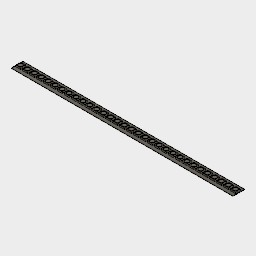
1376 NeoPixel Strip [parametric] (Autodesk Fusion 360 design; units mm, degrees)
Autodesk Fusion 360 part; units mm, degrees
sketch "pixels" plane through (0, 0, 0) normal (0, 0, 1) x (1, 0, 0)
  line L0 (0, 0) -> (224, 0)
  line L1 (224, 0) -> (224, 12)
  line L2 (224, 12) -> (0, 12)
  line L3 (0, 12) -> (0, 0)
  line L4 (0, 6) -> (224, 6) construction
  line L5 (6, 3.5) -> (1, 3.5)
  line L6 (1, 3.5) -> (1, 8.5)
  line L7 (1, 8.5) -> (6, 8.5)
  line L8 (6, 8.5) -> (6, 3.5)
  line L9 (6, 3.5) -> (1, 8.5) construction
  line L10 (1, 3.5) -> (6, 8.5) construction
  line L11 (13, 3.5) -> (8, 3.5)
  line L12 (8, 3.5) -> (8, 8.5)
  line L13 (8, 8.5) -> (13, 8.5)
  line L14 (13, 8.5) -> (13, 3.5)
  line L15 (20, 3.5) -> (15, 3.5)
  line L16 (15, 3.5) -> (15, 8.5)
  line L17 (15, 8.5) -> (20, 8.5)
  line L18 (20, 8.5) -> (20, 3.5)
  line L19 (27, 3.5) -> (22, 3.5)
  line L20 (22, 3.5) -> (22, 8.5)
  line L21 (22, 8.5) -> (27, 8.5)
  line L22 (27, 8.5) -> (27, 3.5)
  line L23 (34, 3.5) -> (29, 3.5)
  line L24 (29, 3.5) -> (29, 8.5)
  line L25 (29, 8.5) -> (34, 8.5)
  line L26 (34, 8.5) -> (34, 3.5)
  line L27 (41, 3.5) -> (36, 3.5)
  line L28 (36, 3.5) -> (36, 8.5)
  line L29 (36, 8.5) -> (41, 8.5)
  line L30 (41, 8.5) -> (41, 3.5)
  line L31 (48, 3.5) -> (43, 3.5)
  line L32 (43, 3.5) -> (43, 8.5)
  line L33 (43, 8.5) -> (48, 8.5)
  line L34 (48, 8.5) -> (48, 3.5)
  line L35 (55, 3.5) -> (50, 3.5)
  line L36 (50, 3.5) -> (50, 8.5)
  line L37 (50, 8.5) -> (55, 8.5)
  line L38 (55, 8.5) -> (55, 3.5)
  line L39 (62, 3.5) -> (57, 3.5)
  line L40 (57, 3.5) -> (57, 8.5)
  line L41 (57, 8.5) -> (62, 8.5)
  line L42 (62, 8.5) -> (62, 3.5)
  line L43 (69, 3.5) -> (64, 3.5)
  line L44 (64, 3.5) -> (64, 8.5)
  line L45 (64, 8.5) -> (69, 8.5)
  line L46 (69, 8.5) -> (69, 3.5)
  line L47 (76, 3.5) -> (71, 3.5)
  line L48 (71, 3.5) -> (71, 8.5)
  line L49 (71, 8.5) -> (76, 8.5)
  line L50 (76, 8.5) -> (76, 3.5)
  line L51 (83, 3.5) -> (78, 3.5)
  line L52 (78, 3.5) -> (78, 8.5)
  line L53 (78, 8.5) -> (83, 8.5)
  line L54 (83, 8.5) -> (83, 3.5)
  line L55 (90, 3.5) -> (85, 3.5)
  line L56 (85, 3.5) -> (85, 8.5)
  line L57 (85, 8.5) -> (90, 8.5)
  line L58 (90, 8.5) -> (90, 3.5)
  line L59 (97, 3.5) -> (92, 3.5)
  line L60 (92, 3.5) -> (92, 8.5)
  line L61 (92, 8.5) -> (97, 8.5)
  line L62 (97, 8.5) -> (97, 3.5)
  line L63 (104, 3.5) -> (99, 3.5)
  line L64 (99, 3.5) -> (99, 8.5)
  line L65 (99, 8.5) -> (104, 8.5)
  line L66 (104, 8.5) -> (104, 3.5)
  line L67 (111, 3.5) -> (106, 3.5)
  line L68 (106, 3.5) -> (106, 8.5)
  line L69 (106, 8.5) -> (111, 8.5)
  line L70 (111, 8.5) -> (111, 3.5)
  line L71 (118, 3.5) -> (113, 3.5)
  line L72 (113, 3.5) -> (113, 8.5)
  line L73 (113, 8.5) -> (118, 8.5)
  line L74 (118, 8.5) -> (118, 3.5)
  line L75 (125, 3.5) -> (120, 3.5)
  line L76 (120, 3.5) -> (120, 8.5)
  line L77 (120, 8.5) -> (125, 8.5)
  line L78 (125, 8.5) -> (125, 3.5)
  line L79 (132, 3.5) -> (127, 3.5)
  line L80 (127, 3.5) -> (127, 8.5)
  line L81 (127, 8.5) -> (132, 8.5)
  line L82 (132, 8.5) -> (132, 3.5)
  line L83 (139, 3.5) -> (134, 3.5)
  line L84 (134, 3.5) -> (134, 8.5)
  line L85 (134, 8.5) -> (139, 8.5)
  line L86 (139, 8.5) -> (139, 3.5)
  line L87 (146, 3.5) -> (141, 3.5)
  line L88 (141, 3.5) -> (141, 8.5)
  line L89 (141, 8.5) -> (146, 8.5)
  line L90 (146, 8.5) -> (146, 3.5)
  line L91 (153, 3.5) -> (148, 3.5)
  line L92 (148, 3.5) -> (148, 8.5)
  line L93 (148, 8.5) -> (153, 8.5)
  line L94 (153, 8.5) -> (153, 3.5)
  line L95 (160, 3.5) -> (155, 3.5)
  line L96 (155, 3.5) -> (155, 8.5)
  line L97 (155, 8.5) -> (160, 8.5)
  line L98 (160, 8.5) -> (160, 3.5)
  line L99 (167, 3.5) -> (162, 3.5)
  line L100 (162, 3.5) -> (162, 8.5)
  line L101 (162, 8.5) -> (167, 8.5)
  line L102 (167, 8.5) -> (167, 3.5)
  line L103 (174, 3.5) -> (169, 3.5)
  line L104 (169, 3.5) -> (169, 8.5)
  line L105 (169, 8.5) -> (174, 8.5)
  line L106 (174, 8.5) -> (174, 3.5)
  line L107 (181, 3.5) -> (176, 3.5)
  line L108 (176, 3.5) -> (176, 8.5)
  line L109 (176, 8.5) -> (181, 8.5)
  line L110 (181, 8.5) -> (181, 3.5)
  line L111 (188, 3.5) -> (183, 3.5)
  line L112 (183, 3.5) -> (183, 8.5)
  line L113 (183, 8.5) -> (188, 8.5)
  line L114 (188, 8.5) -> (188, 3.5)
  line L115 (195, 3.5) -> (190, 3.5)
  line L116 (190, 3.5) -> (190, 8.5)
  line L117 (190, 8.5) -> (195, 8.5)
  line L118 (195, 8.5) -> (195, 3.5)
  line L119 (202, 3.5) -> (197, 3.5)
  line L120 (197, 3.5) -> (197, 8.5)
  line L121 (197, 8.5) -> (202, 8.5)
  line L122 (202, 8.5) -> (202, 3.5)
  line L123 (209, 3.5) -> (204, 3.5)
  line L124 (204, 3.5) -> (204, 8.5)
  line L125 (204, 8.5) -> (209, 8.5)
  line L126 (209, 8.5) -> (209, 3.5)
  line L127 (216, 3.5) -> (211, 3.5)
  line L128 (211, 3.5) -> (211, 8.5)
  line L129 (211, 8.5) -> (216, 8.5)
  line L130 (216, 8.5) -> (216, 3.5)
  line L131 (223, 3.5) -> (218, 3.5)
  line L132 (218, 3.5) -> (218, 8.5)
  line L133 (218, 8.5) -> (223, 8.5)
  line L134 (223, 8.5) -> (223, 3.5)
  point P0 (3.5, 6)
  dimension "d4" = 224
  dimension "d5" = 12
  dimension "d6" = 5
  dimension "d7" = 5
  dimension "d8" = 3.5
  dimension "d11" = 7
  dimension "d12" = 0
  measures "d4" distance of L0.start L0.end
  measures "d5" distance of L0.start L2.end
  measures "d6" distance of L6.end L7.end
  measures "d7" distance of L5.end L6.end
  measures "d8" distance of L3 P0
extrude "Extrude1" add sketch "pixels" along normal blind 0.34 contours L0 L1 L2 L3 | L5 L6 L7 L8 | L11 L12 L13 L14 | L15 L16 L17 L18 | L19 L20 L21 L22 | L23 L24 L25 L26 | L27 L28 L29 L30 | L31 L32 L33 L34 | L35 L36 L37 L38 | L39 L40 L41 L42 | L43 L44 L45 L46 | L47 L48 L49 L50 | L51 L52 L53 L54 | L55 L56 L57 L58 | L59 L60 L61 L62 | L63 L64 L65 L66 | L67 L68 L69 L70 | L71 L72 L73 L74 | L75 L76 L77 L78 | L79 L80 L81 L82 | L83 L84 L85 L86 | L87 L88 L89 L90 | L91 L92 L93 L94 | L95 L96 L97 L98 | L99 L100 L101 L102 | L103 L104 L105 L106 | L107 L108 L109 L110 | L111 L112 L113 L114 | L115 L116 L117 L118 | L119 L120 L121 L122 | L123 L124 L125 L126 | L127 L128 L129 L130 | L131 L132 L133 L134
extrude "Extrude2" add sketch "pixels" along normal blind 1.4 from surface at 0.34 contours L5 L6 L7 L8
pattern_linear "R-Pattern2" count 32 spacing 7 along (1, 0, 0) of "Extrude2"
sketch "circles" plane through (0, 0, 1.74) normal (0, 0, 1) x (-1, 0, 0)
  line L0 (-6, -8.5) -> (-1, -8.5)
  line L1 (-1, -8.5) -> (-1, -3.5)
  line L2 (-1, -3.5) -> (-6, -3.5)
  line L3 (-6, -3.5) -> (-6, -8.5)
  line L4 (-1, -6) -> (-6, -6) construction
  line L5 (-3.5, -8.5) -> (-3.5, -3.5) construction
  circle A0 centre (-3.5, -6) radius 2
  dimension "d20" = 4
  measures "d20" diameter of A0
extrude "Extrude3" cut sketch "circles" against normal blind 0.2 contours A0
pattern_linear "R-Pattern1" count 32 spacing 7 along (1, 0, 0) of "Extrude3"
equation "width = 12 mm"
equation "thickness = 0.34 mm"
equation "pixels = 32"
equation "d4 = pixels * pitch"
equation "d5 = width"
equation "d8 = pitch / 2"
equation "d9 = pixels"
equation "d11 = pitch"
equation "d13 = thickness"
equation "d21 = pixels"
equation "d23 = -pitch"
equation "pitch = 7 mm"
equation "d30 = pixels"
equation "d32 = -pitch"
named bodies: "neostrip"
